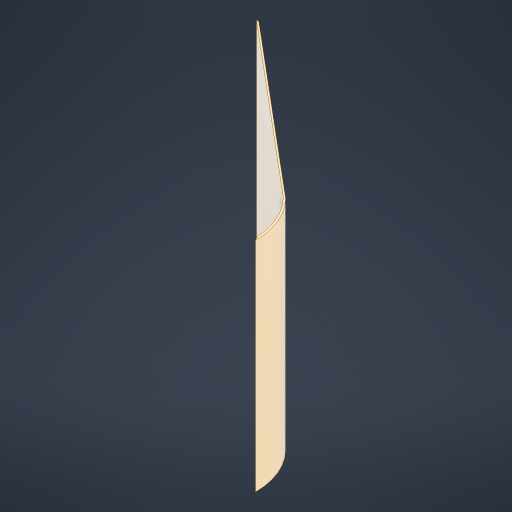
# Autodesk Inventor part: intakeabs
Saved by Autodesk Inventor 2023 (Build 270158000, 158)
## iProperties
Created: 2023-02-25
Part Number: intakeabs
Material: Polyethylene, High Density
Document SubType Name: Modeling
Designer: Windows Macbook
Density: 0.952 g/cm^3
Appearance: Smooth - Off-White
Author: Windows Macbook
Autodesk Inventor part; units mm, degrees
ref_plane "YZ Plane" through (0, 0, 0) normal (1, 0, 0) x (0, 1, 0)
ref_plane "XZ Plane" through (0, 0, 0) normal (0, 1, 0) x (-1, 0, 0)
ref_plane "XY Plane" through (0, 0, 0) normal (0, 0, 1) x (1, 0, 0)
sketch "Sketch1" plane through (0, 0, 0) normal (0, 1, 0) x (-1, 0, 0)
  line L0 (0, 0) -> (203.2, 0) construction
  arc A0 (0, 0) -> (14.879, -35.921) centre (50.8, 0) ccw
  line L1 (14.879, -35.921) -> (192.679, -35.921) construction
  line L2 (14.879, -35.921) -> (131.6241, -133.8819)
  line L3 (14.879, -35.921) -> (167.279, -35.921) construction
  line L4 (16.4665, -35.921) -> (133.2116, -133.8819)
  line L5 (0, 0) -> (1.6699, -2.8924)
  line L6 (0, 0) -> (3.3398, 0) construction
  arc A1 (1.6699, -2.8924) -> (16.4665, -35.921) centre (52.3875, 0) ccw
  line L7 (131.6241, -133.8819) -> (133.2116, -133.8819)
  dimension "d5" = 152.4
  dimension "d6" = 40
  dimension "d7" = 152.4
  dimension "d8" = 60
  constraints: 16 end point, 5 horizontal, 4 point on circle, 2 centre point, 2 equal length
  measures "d5" distance of L1.start L2.end
  measures "d6" angle of L2 L3
  measures "d7" distance of L4.start L4.end
  measures "d8" angle of L5 L6
extrude "Extrusion1" add sketch "Sketch1" along normal blind 152.4
body "Solid1"
